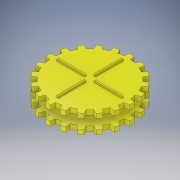
# Autodesk Inventor part: Double cogwheel
Saved by Autodesk Inventor 2018.3 (Build 223284000, 284)
## iProperties
Created: 2020-03-24
Part Number: Double cogwheel
Material: Generic
Document SubType Name: Modeling
Designer: ToreDenStore
Density: 1 g/cm^3
Appearance: Default
Author: ToreDenStore
Autodesk Inventor part; units mm, degrees
ref_plane "YZ Plane" through (0, 0, 0) normal (1, 0, 0) x (0, 1, 0)
ref_plane "XZ Plane" through (0, 0, 0) normal (0, 1, 0) x (-1, 0, 0)
sketch "Sketch1" plane through (0, 0, 0) normal (0, 1, 0) x (-1, 0, 0)
  point P0 (0, 0)
sketch "Sketch2" plane through (0, 0, 0) normal (0, 1, 0) x (-1, 0, 0)
  circle A0 centre (0, 0) radius 40
  line L0 (45, 2.5) -> (45, -2.5)
  line L1 (45, -2.5) -> (39.8546, -3.4073)
  line L2 (45, 2.5) -> (39.8546, 3.4073)
  line L3 (0, 0) -> (45, 0) construction
  dimension "d0" = 80
  dimension "d1" = 5
  dimension "d2" = 100
  dimension "d3" = 100
  dimension "d4" = 2.5
  dimension "d5" = 90
  dimension "d6" = 45
  constraints: 8 end point, 2 point on circle, 1 centre point, 1 coincident, 1 midpoint, 1 vertical
  measures "d0" diameter of A0
  measures "d1" distance of L0.start L0.end
  measures "d2" angle of L1 L0
  measures "d3" angle of L2 L0
  measures "d4" distance of L0.end L3.end
  measures "d5" angle of L0 L3
  measures "d6" distance from line of L0 L3.start
extrude "Extrusion1" add sketch "Sketch2" along normal blind 5
pattern_circular "Circular Pattern1" count 20 over 360 about axis through (0, 0, 0) along (0, 1, 0) of "Extrusion1"
sketch "Sketch3" plane through (0, 5, 0) normal (0, 1, 0) x (1, 0, 0)
  circle A0 centre (0, 0) radius 15
  dimension "d16" = 30
  constraints: 1 centre point, 1 coincident
  measures "d16" diameter of A0
extrude "Extrusion2" add sketch "Sketch3" along normal blind 10
ref_plane "Work Plane1" through (0, 10, 0) normal (0, 1, 0) x (1, 0, 0)
mirror "Mirror1" about plane through (0, 10, 0) normal (0, 1, 0) of "Extrusion1", "Circular Pattern1"
sketch "Sketch4" plane through (-2.5, 20, 45) normal (0, 1, 0) x (1, 0, 0)
  line L0 (37.5, 46) -> (7.5, 46)
  line L1 (7.5, 44) -> (37.5, 44)
  line L2 (7.5, 46) -> (7.5, 44)
  line L3 (37.5, 44) -> (37.5, 46)
  line L4 (2.5, 45) -> (7.5, 45) construction
  dimension "d23" = 5
  dimension "d24" = 30
  dimension "d25" = 2
  dimension "d26" = 1
  dimension "d27" = 90
  dimension "d28" = 90
  constraints: 10 end point, 1 midpoint, 1 parallel, 1 perpendicular
  measures "d23" distance from line of L4.start L2
  measures "d24" distance of L0.start L0.end
  measures "d25" distance of L0.end L1.start
  measures "d26" vertical distance of L4.start L0.end
  measures "d27" angle of L0 L2
  measures "d28" angle of L2 L4
extrude "Extrusion3" add sketch "Sketch4" along normal blind 1
sketch "Sketch6" plane through (35, 20, 1) normal (1, 0, 0) x (0, 0, -1)
  line L0 (2, 0) -> (0, 0) projected
  line L1 (2, 0) -> (2, 1) projected
  line L2 (0, 1) -> (2, 1) construction
  line L3 (0, 0) -> (0, 1) projected
  line L4 (0, 0) -> (0, 1) projected
  line L5 (0, 1) -> (0, 2)
  line L6 (0, 2) -> (2, 2)
  line L7 (2, 2) -> (2, 1)
  point P0 (1, -20)
  dimension "d39" = 1
  constraints: 6 end point, 2 perpendicular, 1 vertical
  measures "d39" distance of L2.start L5.end
extrude "Extrusion4" add sketch "Sketch6" against normal blind 30
sketch "Sketch7" plane through (35, 20, 1) normal (1, 0, 0) x (0, 0, -1)
  line L0 (0, 2) -> (2, 2) projected
  circle A0 centre (1, 2) radius 1
  point P0 (1, -20)
  dimension "d42" = 2
  constraints: 1 centre point, 1 midpoint
  measures "d42" diameter of A0
extrude "Extrusion5" cut sketch "Sketch7" against normal blind 30
pattern_circular "Circular Pattern3" count 4 over 360 about axis through (0, 20, 0) along (0, 1, 0) of "Extrusion3", "Extrusion4", "Extrusion5"
mirror "Mirror2" about plane through (0, 10, 0) normal (0, 1, 0) of "Extrusion3", "Circular Pattern3", "Extrusion4", "Extrusion5"
body "Solid1"
